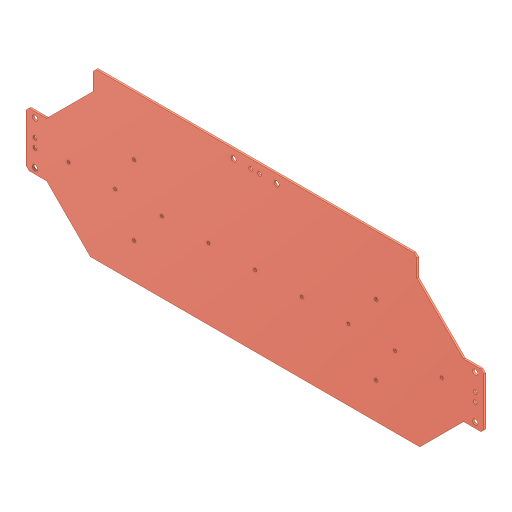
# Autodesk Inventor part: enc - SidePanel Oben V2
Saved by Autodesk Inventor 2023.2 (Build 272271000, 271)
## iProperties
Created: 2023-12-14
Part Number: enc - SidePanel Oben V2
Material: Generisch
Document SubType Name: Modeling
Designer: Nils Bade
Density: 1 g/cm^3
Appearance: PVC Verglasung
Description: Fertigung
Auf Bestellliste: True
Author: Nils Bade
Autodesk Inventor part; units mm, degrees
ref_plane "YZ Plane" through (0, 0, 0) normal (1, 0, 0) x (0, 1, 0)
ref_plane "XZ Plane" through (0, 0, 0) normal (0, 1, 0) x (-1, 0, 0)
ref_plane "XY Plane" through (0, 0, 0) normal (0, 0, 1) x (1, 0, 0)
sketch "Skizze1" plane through (0, 0, 0) normal (0, 0, 1) x (1, 0, 0)
  line L0 (-397.5, 166.5) -> (397.5, 166.5)
  line L1 (397.5, 166.5) -> (397.5, -166.5)
  line L2 (397.5, -166.5) -> (-397.5, -166.5)
  line L3 (-397.5, -166.5) -> (-397.5, 166.5)
  line L4 (-397.5, 166.5) -> (397.5, -166.5) construction
  line L5 (397.5, 166.5) -> (-397.5, -166.5) construction
  line L6 (-357.5, 126.5) -> (357.5, 126.5)
  line L7 (357.5, 126.5) -> (357.5, -126.5)
  line L8 (357.5, -126.5) -> (-357.5, -126.5)
  line L9 (-357.5, -126.5) -> (-357.5, 126.5)
  line L10 (0, 233.1) -> (0, -233.1) construction
  line L11 (-397.5, 46.5) -> (-357.5, 46.5)
  line L12 (-357.5, 46.5) -> (-277.5, 126.5)
  line L13 (-277.5, 126.5) -> (-277.5, 166.5)
  line L14 (-397.5, -46.5) -> (-357.5, -46.5)
  line L15 (-357.5, -46.5) -> (-277.5, -126.5)
  line L16 (-277.5, -126.5) -> (-277.5, -166.5)
  line L17 (357.5, 46.5) -> (277.5, 126.5)
  line L18 (277.5, 126.5) -> (277.5, 166.5)
  line L19 (397.5, -46.5) -> (357.5, -46.5)
  line L20 (357.5, -46.5) -> (277.5, -126.5)
  line L21 (392.5, 161.5) -> (-392.5, 161.5)
  line L22 (-392.5, 161.5) -> (-392.5, -161.5)
  line L23 (-392.5, -161.5) -> (392.5, -161.5)
  line L24 (392.5, -161.5) -> (392.5, 161.5)
  circle A0 centre (-207.5, -60) radius 2.75
  line L25 (-556.5, 0) -> (556.5, 0) construction
  circle A1 centre (-207.5, 60) radius 2.75
  circle A2 centre (207.5, -60) radius 2.75
  circle A3 centre (207.5, 60) radius 2.75
  line L26 (-385.5, -45) -> (-369.5, -45) construction
  line L27 (-369.5, -45) -> (-369.5, 45) construction
  line L28 (-369.5, 45) -> (-385.5, 45) construction
  line L29 (-385.5, 45) -> (-385.5, -45) construction
  line L30 (-385.5, -45) -> (-369.5, 45) construction
  line L31 (-369.5, -45) -> (-385.5, 45) construction
  circle A4 centre (-377.5, -7.5) radius 3.25
  circle A5 centre (-377.5, -37) radius 4.5
  line L32 (-369.5, 0) -> (-385.5, 0) construction
  line L33 (-377.5, -45) -> (-377.5, 45) construction
  circle A6 centre (-377.5, 37) radius 4.5
  circle A7 centre (-377.5, 7.5) radius 3.25
  line L34 (-47.5, 154.5) -> (47.5, 154.5) construction
  line L35 (47.5, 154.5) -> (47.5, 138.5) construction
  line L36 (47.5, 138.5) -> (-47.5, 138.5) construction
  line L37 (-47.5, 138.5) -> (-47.5, 154.5) construction
  line L38 (-47.5, 154.5) -> (47.5, 138.5) construction
  line L39 (47.5, 154.5) -> (-47.5, 138.5) construction
  line L40 (-47.5, 146.5) -> (47.5, 146.5) construction
  circle A8 centre (-7.5, 146.5) radius 3.25
  circle A9 centre (-37, 146.5) radius 4.5
  circle A10 centre (7.5, 146.5) radius 3.25
  circle A11 centre (37, 146.5) radius 4.5
  circle A12 centre (377.5, -37) radius 4.5
  circle A13 centre (377.5, -7.5) radius 3.25
  circle A14 centre (377.5, 7.5) radius 3.25
  circle A15 centre (377.5, 37) radius 4.5
  circle A16 centre (0, 0) radius 2.5
  circle A17 centre (80, 0) radius 2.5
  circle A18 centre (160, 0) radius 2.5
  circle A19 centre (240, 0) radius 2.5
  circle A20 centre (320, 0) radius 2.5
  circle A21 centre (-80, 0) radius 2.5
  circle A22 centre (-160, 0) radius 2.5
  circle A23 centre (-240, 0) radius 2.5
  circle A24 centre (-320, 0) radius 2.5
  line L41 (-282.5, -121.5) -> (282.5, -121.5)
  line L42 (397.5, 46.5) -> (357.5, 46.5)
  line L43 (277.5, -126.5) -> (277.5, -166.5)
  point P0 (0, 0)
  point P1 (277.5, 161.5)
  point P2 (-277.5, 161.5)
  point P3 (-392.5, 46.5)
  point P4 (-392.5, -46.5)
  point P5 (-310.6574, -126.5)
  point P6 (277.5, -126.5)
  point P7 (392.5, -46.5)
  point P8 (-207.5, 0)
  point P9 (-377.5, 0)
  point P10 (0, 146.5)
  point P11 (392.5, 46.5)
  point P12 (277.5, -161.5)
  point P13 (-277.5, -161.5)
  dimension "d0" = 795
  dimension "d1" = 333
  dimension "d2" = 40
  dimension "d13" = 5
  dimension "d16" = 5.5
  dimension "d22" = 60
  dimension "d25" = 16
  dimension "d26" = 90
  dimension "d27" = 6.5
  dimension "d28" = 9
  dimension "d29" = 7.5
  dimension "d30" = 37
  dimension "d33" = 20
  dimension "d34" = 95
  dimension "d35" = 16
  dimension "d36" = 20
  dimension "d37" = 6.5
  dimension "d38" = 9
  dimension "d39" = 7.5
  dimension "d40" = 37
  dimension "d41" = 5
  dimension "d44" = 80
  dimension "d51" = 80
  dimension "d56" = 5
  dimension "d57" = 121.5
  dimension "d58" = 120
  dimension "d59" = 120
  dimension "d60" = 120
  dimension "d61" = 120
  constraints: 84 end point, 25 centre point, 19 symmetric about line, 15 point on line, 12 midpoint, 10 parallel, 6 horizontal, 5 perpendicular, 1 coincident, 1 vertical, 33 other
  measures "d0" distance of L0.start L0.end
  measures "d1" distance of L2.end L0.start
  measures "d2" distance between parallel lines of L3 L9
  measures "d13" distance between parallel lines of L0 L21
  measures "d16" diameter of A0
  measures "d22" distance from line of L25 A0.centre
  measures "d25" distance of L29.start L30.end
  measures "d26" distance of L30.end L26.end
  measures "d27" diameter of A4
  measures "d28" diameter of A5
  measures "d29" distance from line of L32 A4.centre
  measures "d30" distance from line of A5.centre L32
  measures "d33" distance between parallel lines of L3 L33
  measures "d34" distance of L35.end L36.end
  measures "d35" distance of L34.end L35.end
  measures "d36" distance between parallel lines of L0 L40
  measures "d37" diameter of A8
  measures "d38" diameter of A9
  measures "d39" distance from line of L10 A8.centre
  measures "d40" distance from line of L10 A9.centre
  measures "d41" diameter of A16
  measures "d44" distance of A16.centre A17.centre
  measures "d51" distance of A16.centre A21.centre
  measures "d56" distance between parallel lines of L41 L8
  measures "d57" distance between parallel lines of L41 L25
  measures "d58" distance between parallel lines of L3 L13
  measures "d59" distance between parallel lines of L0 L11
  measures "d60" distance between parallel lines of L2 L14
  measures "d61" distance between parallel lines of L3 L16
extrude "Extrusion1" add sketch "Skizze1" along normal blind 3 contours L21 L18 L6 L13 | L11 L9 L14 L22 | L6 L17 L7 L20 L41 L15 L9 L12 | L24 L19 L7 L42
chamfer "Fase-5mm" distance 5 angle 45 6 edges at (-277.5, 161.5, 1.5) (277.5, 161.5, 1.5) (392.5, 46.5, 1.5) (392.5, -46.5, 1.5) (-392.5, -46.5, 1.5) (-392.5, 46.5, 1.5)
equation "\"d37\" = d27"
equation "\"d38\" = d28"
equation "\"d39\" = d29"
equation "\"d40\" = d30"
equation "\"d59\" = d58"
equation "\"d60\" = d58"
equation "\"d61\" = d58"
